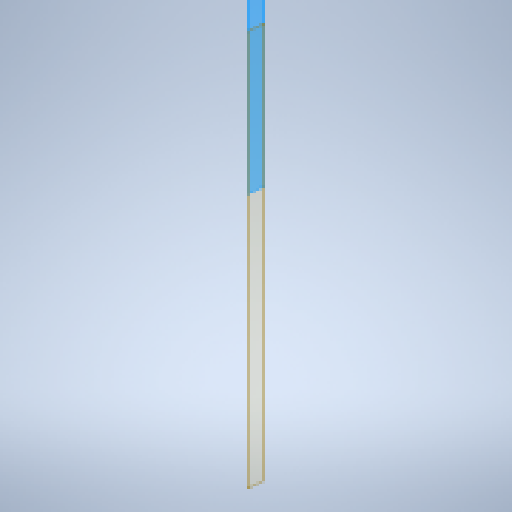
# Autodesk Inventor part: Album
Saved by Autodesk Inventor 2023 (Build 270158000, 158)
## iProperties
Created: 2023-02-02
Part Number: Album
Material: Generic
Document SubType Name: Modeling
Designer: shrey
Density: 1 g/cm^3
Appearance: Default
Author: shrey
Autodesk Inventor part; units mm, degrees
ref_plane "YZ Plane" through (0, 0, 0) normal (1, 0, 0) x (0, 1, 0)
ref_plane "XZ Plane" through (0, 0, 0) normal (0, 1, 0) x (-1, 0, 0)
ref_plane "XY Plane" through (0, 0, 0) normal (0, 0, 1) x (1, 0, 0)
ref_plane "Work Plane2" through (294.5223, -137.0479, 294.5223) normal (0, 0, 1) x (-1, 0, 0)
sketch "Sketch2" plane through (294.5223, -137.0479, 294.5223) normal (0, 0, 1) x (-1, 0, 0)
  line L0 (451.6723, 20.1021) -> (137.3723, 20.1021)
  line L1 (137.3723, 20.1021) -> (137.3723, -294.1979)
  line L2 (137.3723, -294.1979) -> (451.6723, -294.1979)
  line L3 (451.6723, -294.1979) -> (451.6723, 20.1021)
  line L4 (451.6723, 20.1021) -> (137.3723, -294.1979) construction
  line L5 (137.3723, 20.1021) -> (451.6723, -294.1979) construction
  point P0 (294.5223, -137.0479)
  point P1 (294.5223, -137.0479)
  point P2 (294.5223, -137.0479)
  dimension "d0" = 314.3
  dimension "d1" = 314.3
  constraints: 12 end point, 2 midpoint, 2 parallel, 1 coincident, 1 horizontal, 1 perpendicular
  measures "d0" distance of L2.end L1.end
  measures "d1" distance of L0.end L1.end
extrude "Extrusion1" add sketch "Sketch2" along normal blind 10
body "Solid1"
